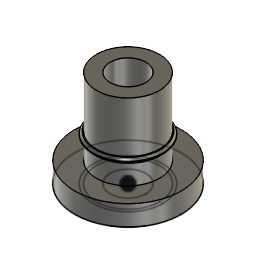
Alfa 147 Handle Saddle (Autodesk Fusion 360 design; units mm, degrees)
Autodesk Fusion 360 part; units mm, degrees
sketch "Sketch1" plane through (0, 0, 0) normal (0, 0, 1) x (1, 0, 0)
  circle A0 centre (0, 0) radius 5.25
  circle A1 centre (0, 0) radius 3.1
  circle A2 centre (0, 0) radius 1.75
  circle A3 centre (0, 0) radius 3.4
  dimension "d1" = 10.5
  dimension "d2" = 6.2
  dimension "d3" = 3.5
  dimension "d8" = 6.8
  constraint coincident A0.centre A1.centre
  constraint concentric A0 A2
  constraint concentric A2 A3
  measures "d1" diameter of A0
  measures "d2" diameter of A1
  measures "d3" diameter of A2
  measures "d8" diameter of A3
extrude "Extrude1" add sketch "Sketch1" along normal blind 9.5 contours A1
extrude "Extrude2" add sketch "Sketch1" along normal blind 2 contours A0 | A3
extrude "Extrude3" add sketch "Sketch1" along normal blind 4 and the other way blind -4.5 contours A3
chamfer "Chamfer1" distance 0.2 angle 45 2 edges at (-3.1699, -1.2295, 4) (-3.1699, -1.2295, 4.5)
chamfer "Chamfer2" distance 0.5 angle 45 1 edges at (-1.6316, 0.6328, 0)
